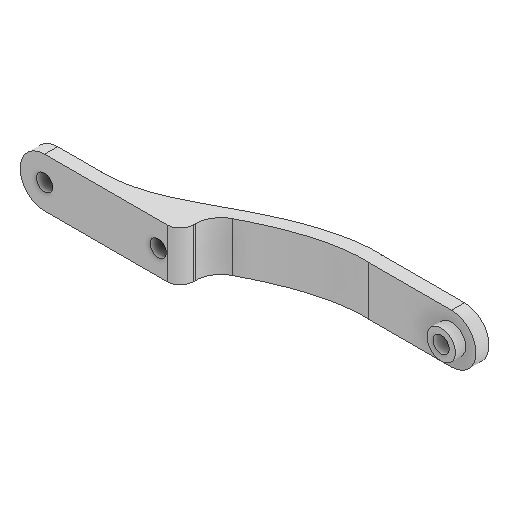
# Autodesk Inventor part: swingarmV1
Saved by Autodesk Inventor 2025 (Build 290162000, 162)
## iProperties
Created: 2024-10-14
Part Number: swingarmV1
Material: Generic
Document SubType Name: Modeling
Designer: derm
Density: 1 g/cm^3
Appearance: Default
Author: derm
Autodesk Inventor part; units mm, degrees
ref_plane "YZ Plane" through (0, 0, 0) normal (1, 0, 0) x (0, 1, 0)
ref_plane "XZ Plane" through (0, 0, 0) normal (0, 1, 0) x (-1, 0, 0)
ref_plane "XY Plane" through (0, 0, 0) normal (0, 0, 1) x (1, 0, 0)
sketch "Sketch1" plane through (0, 0, 0) normal (0, 0, 1) x (1, 0, 0)
  line L0 (0, 0) -> (165.1, 0) construction
  line L1 (0, -11.995) -> (165.1, -11.995)
  line L2 (165.1, 11.995) -> (0, 11.995)
  arc A0 (0, 11.995) -> (0, -11.995) centre (0, 0) ccw
  arc A1 (165.1, -11.995) -> (165.1, 11.995) centre (165.1, 0) ccw
  circle A2 centre (0, 0) radius 4
  circle A3 centre (165.1, 0) radius 4
  point P0 (82.55, 0)
  dimension "d0" = 165.1
  dimension "d1" = 8
  dimension "d2" = 8
  constraints: 8 end point, 4 centre point, 4 point on circle, 4 tangent, 2 coincident, 1 horizontal, 1 midpoint, 1 parallel
  measures "d0" distance of L0.start L0.end
  measures "d1" diameter of A3
  measures "d2" diameter of A2
extrude "Extrusion1" add sketch "Sketch1" along normal blind 6.35
sketch "Sketch2" plane through (0, 0, 6.35) normal (0, 0, 1) x (1, 0, 0)
  circle A0 centre (165.1, 0) radius 4 projected
  arc A1 (165.1, -11.995) -> (165.1, 11.995) centre (165.1, 0) ccw projected
  circle A2 centre (165.1, 0) radius 7
  point P0 (0, 0)
  dimension "d5" = 14
  constraints: 1 centre point, 1 coincident
  measures "d5" diameter of A2
extrude "Extrusion2" add sketch "Sketch2" along normal blind 5
ref_plane "Work Plane1" through (0, 0, 39.624) normal (0, 0, 1) x (1, 0, 0)
sketch "Sketch3" plane through (0, 0, 39.624) normal (0, 0, 1) x (1, 0, 0)
  circle A0 centre (165.1, 0) radius 7 projected
  arc A1 (165.1, -11.995) -> (165.1, 11.995) centre (165.1, 0) ccw projected
  line L0 (165.1, 11.995) -> (0, 11.995) projected
  arc A2 (0, 11.995) -> (0, -11.995) centre (0, 0) ccw projected
  line L1 (0, -11.995) -> (165.1, -11.995) projected
  circle A3 centre (0, 0) radius 4 projected
  line L2 (21.4998, 18.3449) -> (21.4998, -29.3285)
  point P0 (21.4998, -11.995)
  point P1 (21.4998, 11.995)
  constraints: 2 end point, 1 vertical
extrude "Extrusion3" add sketch "Sketch3" against normal blind 6.35 contours L1 A2 L0 L2
sketch "Sketch4" plane through (0, 0, 0) normal (0, 0, -1) x (-1, 0, 0)
  line L0 (60.3594, -52.6413) -> (-124.8747, -52.6413)
  line L1 (-124.8747, -52.6413) -> (-124.8747, 49.8707)
  line L2 (-124.8747, 49.8707) -> (60.3594, 49.8707)
  line L3 (60.3594, 49.8707) -> (60.3594, -52.6413)
  point P0 (0, 0)
  constraints: 8 end point, 2 parallel, 1 horizontal, 1 perpendicular
extrude "Extrusion4" cut sketch "Sketch4" against normal blind 10
ref_plane "Work Plane2" through (0, 0, 39.624) normal (0, -1, 0) x (1, 0, 0)
sketch "Sketch5" plane through (0, 0, 39.624) normal (0, -1, 0) x (1, 0, 0)
  line L0 (21.4998, 0) -> (21.4998, -6.35) projected
  line L1 (21.4998, -3.175) -> (52.8311, -3.175) construction
  line L2 (52.8311, -3.175) -> (66.153, -23.1563) construction
  line L3 (66.153, -23.1563) -> (101.0317, -37.8743) construction
  line L4 (124.8747, -33.274) -> (124.8747, -39.624) projected
  line L5 (101.0317, -37.8743) -> (124.8747, -36.449) construction
  spline S0 degree 4 poles (21.4998, -3.175) (52.8311, -3.175) (66.153, -23.1563) (101.0317, -37.8743) (124.8747, -36.449) knots 1 1 1 1 1 2 2 2 2 2
  line L6 (124.8747, -36.449) -> (128.9819, -36.449)
  point P0 (0, -39.624)
  constraints: 2 end point, 2 horizontal, 2 midpoint, 3 other
sketch "Sketch6" plane through (21.4998, -11.995, 39.624) normal (1, 0, 0) x (0, 0, -1)
  line L0 (0, 0) -> (0, 23.9899) projected
  line L1 (0, 0) -> (6.35, 0) projected
  line L2 (6.35, 23.9899) -> (6.35, 0) projected
  line L3 (0, 23.9899) -> (6.35, 23.9899) projected
  point P0 (39.624, 11.995)
sweep "Sweep1" add profiles "Sketch6" path "Sketch5" keep normal constant yes path curves S0
sketch "Sketch7" plane through (0, 0, 39.624) normal (0, 0, 1) x (1, 0, 0)
  line L0 (21.4998, -11.995) -> (21.4998, 11.995) projected
  line L1 (21.4998, -11.995) -> (124.8747, -11.995) projected
  line L2 (124.8747, 11.995) -> (124.8747, -11.995) projected
  line L3 (21.4998, 11.995) -> (124.8747, 11.995) projected
  circle A0 centre (165.1, 0) radius 7 projected
  circle A1 centre (55.4336, 0) radius 4
  line L4 (44.7246, 11.995) -> (66.1427, 11.995)
  line L5 (66.1427, 11.995) -> (66.1427, -11.995)
  line L6 (66.1427, -11.995) -> (44.7246, -11.995)
  line L7 (44.7246, -11.995) -> (44.7246, 11.995)
  line L8 (44.7246, 11.995) -> (66.1427, -11.995) construction
  line L9 (66.1427, 11.995) -> (44.7246, -11.995) construction
  point P0 (0, 0)
  dimension "d21" = 8
  constraints: 12 end point, 2 midpoint, 2 parallel, 1 centre point, 1 horizontal, 1 perpendicular, 1 point on line
  measures "d21" diameter of A1
extrude "Extrusion5" add sketch "Sketch7" against normal up to next contours L0 L3 L7 L1 | L7 L3 L5 L1
sketch "Sketch8" plane through (0, 0, 39.624) normal (0, 0, 1) x (1, 0, 0)
  circle A0 centre (55.4336, 0) radius 4 projected
  point P0 (0, 0)
extrude "Extrusion6" cut sketch "Sketch8" against normal blind 25.4
ref_plane "Work Plane3" through (0, 0, 26.924) normal (0, 0, 1) x (1, 0, 0)
sketch "Sketch9" plane through (0, 0, 26.924) normal (0, 0, 1) x (1, 0, 0)
  spline S0 degree 2 poles (59.4336, 0) (59.4336, 6.9282) (53.4336, 3.4641) (47.4336, 0) (53.4336, -3.4641) (59.4336, -6.9282) (59.4336, 0) knots 0 0 0 0.333333 0.333333 0.666667 0.666667 1 1 1 weights 1 0.5 1 0.5 1 0.5 1 projected
  circle A0 centre (55.4336, 0) radius 4 projected
  circle A1 centre (55.4336, 0) radius 6.35
  point P0 (0, 0)
  dimension "d20" = 12.7
  constraints: 1 centre point, 1 coincident, 2 other
  measures "d20" diameter of A1
extrude "Extrusion7" cut sketch "Sketch9" against normal blind 25.4
fillet "Fillet1" radius 12.7 1 edges at (66.1427, 0, 24.6668)
fillet "Fillet2" radius 6.35 1 edges at (66.1427, 0, 39.624)
body "Solid1"
